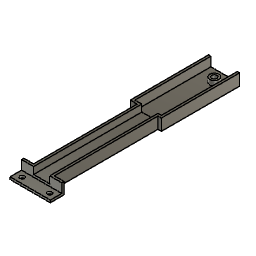
platform_upper (Autodesk Fusion 360 design; units mm, degrees)
Autodesk Fusion 360 part; units mm, degrees
sketch "スケッチ1" plane through (0, 0, 0) normal (0, 0, 1) x (1, 0, 0)
  line L0 (-17.5, 170) -> (17.5, 170)
  line L1 (17.5, 170) -> (17.5, 0)
  line L2 (17.5, 0) -> (-17.5, 0)
  line L3 (-17.5, 0) -> (-17.5, 170)
  circle A0 centre (12, 5) radius 2
  circle A1 centre (-12, 5) radius 2
  line L4 (12, 5) -> (-12, 5) construction
  circle A2 centre (0, 160) radius 2.25
  dimension "d1" = 170
  dimension "d2" = 35
  dimension "d3" = 4
  dimension "d4" = 4
  dimension "d5" = 24
  dimension "d6" = 5
  dimension "d7" = 5.5
  dimension "d8" = 4.5
  dimension "d9" = 155
  constraint horizontal L0
  constraint vertical L1
  constraint horizontal L2
  constraint vertical L3
  constraint midpoint origin L2
  constraint coincident A0.centre L4.start
  constraint coincident A1.centre L4.end
  constraint perpendicular L1 L4
  measures "d1" distance of L0.end L1.end
  measures "d2" distance of L1.end L2.end
  measures "d3" diameter of A0
  measures "d4" diameter of A1
  measures "d5" distance of A0.centre A1.centre
  measures "d6" distance of L2 L4
  measures "d7" distance of L1 A0.centre
  measures "d8" diameter of A2
  measures "d9" distance of L4 A2.centre
extrude "押し出し1" add sketch "スケッチ1" along normal blind 2 makes body 1
sketch "スケッチ2" plane through (0, 0, 2) normal (0, 0, 1) x (-1, 0, 0)
  circle A0 centre (-12, -5) radius 2
  circle A1 centre (0, -160) radius 2.25
  circle A2 centre (12, -5) radius 2
  line L0 (17.5, 0) -> (-17.5, 0)
  line L1 (-17.5, 0) -> (-17.5, -170)
  line L2 (-17.5, -170) -> (17.5, -170)
  line L3 (17.5, -170) -> (17.5, 0)
  line L4 (-7, -170) -> (-17.5, -170)
  line L5 (-17.5, -170) -> (-17.5, -10)
  line L6 (-17.5, -10) -> (-7, -10)
  line L7 (-7, -10) -> (-7, -170)
  line L8 (17.5, -170) -> (7, -170)
  line L9 (7, -170) -> (7, -10)
  line L10 (7, -10) -> (17.5, -10)
  line L11 (17.5, -10) -> (17.5, -170)
  dimension "d12" = 10.5
  dimension "d13" = 10
  dimension "d14" = 10.5
  dimension "d15" = 10
  constraint horizontal L4
  constraint vertical L5
  constraint horizontal L6
  constraint vertical L7
  constraint coincident L1 L5.end
  constraint coincident L2 L4.start
  constraint horizontal L8
  constraint vertical L9
  constraint horizontal L10
  constraint vertical L11
  constraint coincident L2.end L3.start
  measures "d12" distance of L4.start L1.end
  measures "d13" distance of L0 L6
  measures "d14" distance of L2.end L8.end
  measures "d15" distance of L0 L10
extrude "押し出し2" cut sketch "スケッチ2" against normal blind 2 contours L2 L3 L8 L9 L10 L11 | L1 L2 L4 L5 L6 L7 bodies 1
sketch "スケッチ3" plane through (7, 0, 0) normal (1, 0, 0) x (0, 1, 0)
  line L0 (170, 2) -> (10, 2)
  line L1 (10, 2) -> (10, 0)
  line L2 (10, 0) -> (170, 0)
  line L3 (170, 0) -> (170, 2)
  line L4 (10, 10) -> (104, 10)
  line L5 (104, 10) -> (104, 0)
  line L6 (104, 0) -> (10, 0)
  line L7 (10, 0) -> (10, 10)
  dimension "d18" = 10
  dimension "d19" = 94
  constraint horizontal L4
  constraint vertical L5
  constraint horizontal L6
  constraint vertical L7
  constraint coincident L2 L5.end
  constraint collinear L1 L7
  measures "d18" distance of L4.start L1.end
  measures "d19" distance of L4.start L4.end
extrude "押し出し3" add sketch "スケッチ3" along normal blind 2 separate body contours L0 L1 L2 L5 L6 L7 | L0 L4 L5 L7 makes body 2
sketch "スケッチ4" plane through (-7, 0, 0) normal (-1, 0, 0) x (0, -1, 0)
  line L0 (-10, 2) -> (-170, 2)
  line L1 (-170, 2) -> (-170, 0)
  line L2 (-170, 0) -> (-10, 0)
  line L3 (-10, 0) -> (-10, 2)
  line L4 (-10, 10) -> (-104, 10)
  line L5 (-104, 10) -> (-104, 0)
  line L6 (-104, 0) -> (-10, 0)
  line L7 (-10, 0) -> (-10, 10)
  line L8 (-104, 10) -> (-104, 0)
  line L9 (-10, 0) -> (-10, 10)
  line L10 (-10, 10) -> (-104, 10)
  constraint horizontal L4
  constraint vertical L5
  constraint horizontal L6
  constraint vertical L7
  constraint coincident L2 L5.end
  constraint collinear L5 L8
  constraint collinear L7 L9
  constraint collinear L4 L10
extrude "押し出し4" add sketch "スケッチ4" along normal blind 2 separate body contours L0 L2 L3 L5 L6 L7 L8 L9 | L0 L4 L5 L7 L8 L9 L10 makes body 3
sketch "スケッチ5" plane through (0, 0, 2) normal (0, 0, 1) x (-1, 0, 0)
  line L0 (7, -170) -> (7, -10)
  line L1 (7, -10) -> (17.5, -10)
  line L2 (17.5, -10) -> (17.5, 0)
  line L3 (17.5, 0) -> (-17.5, 0)
  line L4 (-17.5, 0) -> (-17.5, -10)
  line L5 (-17.5, -10) -> (-7, -10)
  line L6 (-7, -10) -> (-7, -170)
  line L7 (-7, -170) -> (7, -170)
  circle A0 centre (12, -5) radius 2
  circle A1 centre (0, -160) radius 2.25
  circle A2 centre (-12, -5) radius 2
  line L8 (-7, -170) -> (-10, -170)
  line L9 (-10, -170) -> (-10, -104)
  line L10 (-10, -104) -> (-7, -104)
  line L11 (-7, -104) -> (-7, -170)
  line L12 (-7, -104) -> (-9, -104)
  line L13 (7, -170) -> (13, -170)
  line L14 (13, -170) -> (13, -104)
  line L15 (13, -104) -> (7, -104)
  line L16 (7, -104) -> (7, -170)
  line L17 (7, -104) -> (9, -104)
  dimension "d24" = 3
  dimension "d25" = 6
  constraint horizontal L8
  constraint vertical L9
  constraint horizontal L10
  constraint vertical L11
  constraint coincident L6 L7.start
  constraint collinear L10 L12
  constraint collinear L7 L8
  constraint horizontal L13
  constraint vertical L14
  constraint horizontal L15
  constraint vertical L16
  constraint coincident L0.start L7.end
  constraint collinear L15 L17
  measures "d24" distance of L6.end L8.end
  measures "d25" distance of L0.start L13.end
extrude "押し出し5" add sketch "スケッチ5" against normal blind 2 contours L0 L13 L14 L15 L16 L17 | L6 L8 L9 L10 L11 L12 bodies 1 2 3
sketch "スケッチ10" plane through (-13, 0, 0) normal (-1, 0, 0) x (0, -1, 0)
  line L0 (-104, 2) -> (-170, 2)
  line L1 (-170, 2) -> (-170, 0)
  line L2 (-170, 0) -> (-104, 0)
  line L3 (-104, 0) -> (-104, 2)
  line L4 (-104, 0) -> (-170, 0)
  line L5 (-170, 0) -> (-170, 10)
  line L6 (-170, 10) -> (-104, 10)
  line L7 (-104, 10) -> (-104, 0)
  point P0 (-104, 10)
  constraint horizontal L4
  constraint vertical L5
  constraint horizontal L6
  constraint vertical L7
  constraint coincident L2.end L3.start
  constraint coincident L1.end L5
  constraint coincident L6 P0
extrude "押し出し8" add sketch "スケッチ10" along normal blind 2 separate body makes body 4
sketch "スケッチ11" plane through (10, 0, 0) normal (1, 0, 0) x (0, 1, 0)
  line L0 (170, 2) -> (104, 2)
  line L1 (104, 2) -> (104, 0)
  line L2 (104, 0) -> (170, 0)
  line L3 (170, 0) -> (170, 2)
  line L4 (104, 0) -> (170, 0)
  line L5 (170, 0) -> (170, 10)
  line L6 (170, 10) -> (104, 10)
  line L7 (104, 10) -> (104, 0)
  line L8 (104, 10) -> (10, 10)
  constraint horizontal L4
  constraint vertical L5
  constraint horizontal L6
  constraint vertical L7
  constraint coincident L1.end L2.start
  constraint coincident L2.end L5
  constraint collinear L6 L8
extrude "押し出し9" add sketch "スケッチ11" along normal blind 2 separate body makes body 5
sketch "スケッチ12" plane through (0, 104, 0) normal (0, -1, 0) x (1, 0, 0)
  line L0 (-13, 0) -> (-13, 10)
  line L1 (-13, 10) -> (-15, 10)
  line L2 (-15, 10) -> (-15, 0)
  line L3 (-15, 0) -> (-13, 0)
  line L4 (-15, 10) -> (-7, 10)
  line L5 (-7, 10) -> (-7, 0)
  line L6 (-7, 0) -> (-15, 0)
  line L7 (-15, 0) -> (-15, 10)
  line L8 (-7, 2) -> (-7, 10)
  line L9 (17.5, 0) -> (-17.5, 0)
  line L10 (7, 10) -> (12, 10)
  line L11 (12, 10) -> (12, 0)
  line L12 (12, 0) -> (7, 0)
  line L13 (7, 0) -> (7, 10)
  line L14 (12, 10) -> (12, 0)
  line L15 (7, 2) -> (7, 10)
  line L16 (10, 10) -> (12, 10)
  constraint horizontal L4
  constraint vertical L5
  constraint horizontal L6
  constraint vertical L7
  constraint coincident L1.end L2.start
  constraint collinear L5 L8
  constraint collinear L6 L9
  constraint horizontal L10
  constraint vertical L11
  constraint horizontal L12
  constraint vertical L13
  constraint collinear L11 L14
  constraint collinear L9 L12
  constraint collinear L13 L15
  constraint collinear L10 L16
extrude "押し出し10" add sketch "スケッチ12" along normal blind 2 bodies 1 4 5
sketch "スケッチ13" plane through (0, 10, 0) normal (0, 1, 0) x (-1, 0, 0)
  line L0 (-9, 0) -> (-9, 2)
  line L1 (-9, 2) -> (-17.5, 2)
  line L2 (-17.5, 2) -> (-17.5, 0)
  line L3 (-17.5, 0) -> (-9, 0)
  line L4 (-17.5, 0) -> (-7, 0)
  line L5 (-7, 0) -> (-7, 10)
  line L6 (-7, 10) -> (-17.5, 10)
  line L7 (-17.5, 10) -> (-17.5, 0)
  line L8 (7, 10) -> (17.5, 10)
  line L9 (17.5, 10) -> (17.5, 0)
  line L10 (17.5, 0) -> (7, 0)
  line L11 (7, 0) -> (7, 10)
  point P0 (-7, 10)
  point P1 (7, 10)
  point P2 (17.5, 0)
  constraint horizontal L4
  constraint vertical L5
  constraint horizontal L6
  constraint vertical L7
  constraint coincident L2.end L3.start
  constraint coincident P0 L5.end
  constraint horizontal L8
  constraint vertical L9
  constraint horizontal L10
  constraint vertical L11
  constraint coincident L11 P1
  constraint coincident L8 P1
  constraint coincident L10 P2
  constraint coincident L9 P2
extrude "押し出し11" add sketch "スケッチ13" along normal blind 2 bodies 1
sketch "スケッチ14" plane through (0, 0, 2) normal (0, 0, 1) x (-1, 0, 0)
  line L0 (7, -104) -> (7, -10)
  line L1 (7, -10) -> (17.5, -10)
  line L2 (17.5, -10) -> (17.5, 0)
  line L3 (17.5, 0) -> (-17.5, 0)
  line L4 (-17.5, 0) -> (-17.5, -10)
  line L5 (-17.5, -10) -> (-7, -10)
  line L6 (-7, -10) -> (-7, -104)
  line L7 (-7, -104) -> (-10, -104)
  line L8 (-10, -104) -> (-10, -170)
  line L9 (-10, -170) -> (13, -170)
  line L10 (13, -170) -> (13, -104)
  line L11 (13, -104) -> (7, -104)
  circle A0 centre (12, -5) radius 2
  circle A1 centre (0, -160) radius 2.25
  circle A2 centre (-12, -5) radius 2
  line L12 (7, -104) -> (-7, -104)
  line L13 (-7, -104) -> (-7, -10)
  line L14 (-7, -10) -> (7, -10)
  line L15 (7, -10) -> (7, -104)
  constraint horizontal L12
  constraint vertical L13
  constraint horizontal L14
  constraint vertical L15
  constraint coincident L6 L5.end
  constraint coincident L0 L11.end
  constraint collinear L7 L12
  constraint collinear L5 L14
extrude "押し出し12" add sketch "スケッチ14" along normal blind 2 contours L0 L6 L12 L13 L14 L15 bodies 1
sketch "スケッチ15" plane through (0, 0, 2) normal (0, 0, 1) x (-1, 0, 0)
  circle A0 centre (0, -160) radius 2.25
  line L0 (13, -104) -> (-10, -104)
  line L1 (-10, -104) -> (-10, -170)
  line L2 (-10, -170) -> (13, -170)
  line L3 (13, -170) -> (13, -104)
  circle A1 centre (0, -160) radius 4
  dimension "d43" = 8
  constraint concentric A0 A1
  measures "d43" diameter of A1
extrude "押し出し13" add sketch "スケッチ15" along normal blind 4 contours A1 bodies 1
